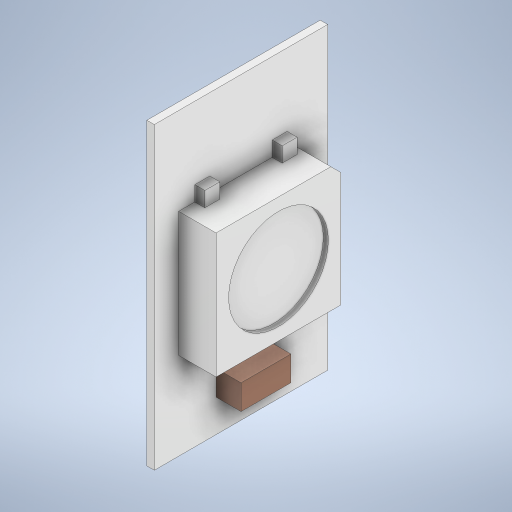
# Autodesk Inventor part: Base144
Saved by Autodesk Inventor 2023 (Build 270158000, 158)
## iProperties
Created: 2024-03-20
Part Number: Base144
Material: Generic
Document SubType Name: Modeling
Designer: noname
Density: 1 g/cm^3
Appearance: Smooth - White
Author: noname
Autodesk Inventor part; units mm, degrees
ref_plane "YZ Plane" through (0, 0, 0) normal (1, 0, 0) x (0, 1, 0)
ref_plane "XZ Plane" through (0, 0, 0) normal (0, 1, 0) x (-1, 0, 0)
ref_plane "XY Plane" through (0, 0, 0) normal (0, 0, 1) x (1, 0, 0)
sketch "Sketch1" plane through (0, 0, 0) normal (1, 0, 0) x (0, 1, 0)
  line L0 (0, 0) -> (12, 0)
  line L1 (12, 0) -> (12, -6.95)
  line L2 (12, -6.95) -> (0, -6.95)
  line L3 (0, -6.95) -> (0, 0)
  dimension "d0" = 12
  dimension "d1" = 6.95
  constraints: 8 end point, 2 parallel, 1 horizontal, 1 perpendicular
  measures "d0" distance between parallel lines of L3 L1
  measures "d1" distance between parallel lines of L2 L0
extrude "Extrusion1" add sketch "Sketch1" along normal blind 0.3
sketch "Sketch2" plane through (0.3, 0, 0) normal (1, 0, 0) x (0, 0, -1)
  line L0 (0.975, 3.5) -> (5.975, 3.5)
  line L1 (5.975, 3.5) -> (5.975, 8.5)
  line L2 (5.975, 8.5) -> (0.975, 8.5)
  line L3 (0.975, 8.5) -> (0.975, 3.5)
  line L4 (6.95, 12) -> (0, 12) projected
  line L5 (6.95, 0) -> (6.95, 12) projected
  point P0 (0, 0)
  point P1 (3.475, 8.5)
  point P2 (3.475, 12)
  point P3 (5.975, 6)
  point P4 (6.95, 6)
  dimension "d4" = 5
  dimension "d5" = 5
  constraints: 8 end point, 4 midpoint, 2 parallel, 1 horizontal, 1 horizontal alignment, 1 perpendicular, 1 vertical alignment
  measures "d4" distance between parallel lines of L1 L3
  measures "d5" distance between parallel lines of L0 L2
extrude "Extrusion2" add sketch "Sketch2" along normal blind 1.5
sketch "Sketch3" plane through (1.8, 0, 0) normal (1, 0, 0) x (0, 0, -1)
  circle A0 centre (3.475, 6) radius 2
  line L0 (0.975, 3.5) -> (5.975, 3.5) projected
  line L1 (5.975, 3.5) -> (5.975, 8.5) projected
  point P0 (0, 0)
  point P1 (3.475, 3.5)
  point P2 (5.975, 6)
  dimension "d8" = 4
  constraints: 2 midpoint, 1 centre point, 1 horizontal alignment, 1 vertical alignment
  measures "d8" diameter of A0
extrude "Extrusion3" cut sketch "Sketch3" against normal blind 0.2
chamfer "Chamfer1" distance 0.4 angle 45 1 edges at (1.05, 8.5, -5.975)
sketch "Sketch5" plane through (0.3, 0, 0) normal (1, 0, 0) x (0, 0, -1)
  line L0 (5.975, 3.5) -> (0.975, 3.5) projected
  line L1 (1.625, 3.5) -> (2.225, 3.5)
  line L2 (2.225, 3.5) -> (2.225, 2.9)
  line L3 (2.225, 2.9) -> (1.625, 2.9)
  line L4 (1.625, 2.9) -> (1.625, 3.5)
  line L5 (0.975, 3.5) -> (0.975, 8.5) projected
  line L6 (0.975, 6) -> (5.975, 6)
  line L7 (5.975, 8.1) -> (5.975, 3.5) projected
  line L8 (3.475, 3.5) -> (3.475, 8.5)
  line L9 (0.975, 8.5) -> (5.575, 8.5) projected
  line L10 (5.325, 3.5) -> (4.725, 3.5)
  line L11 (4.725, 3.5) -> (4.725, 2.9)
  line L12 (4.725, 2.9) -> (5.325, 2.9)
  line L13 (5.325, 2.9) -> (5.325, 3.5)
  line L14 (1.625, 8.5) -> (2.225, 8.5)
  line L15 (2.225, 8.5) -> (2.225, 9.1)
  line L16 (2.225, 9.1) -> (1.625, 9.1)
  line L17 (1.625, 9.1) -> (1.625, 8.5)
  line L18 (5.325, 8.5) -> (4.725, 8.5)
  line L19 (4.725, 8.5) -> (4.725, 9.1)
  line L20 (4.725, 9.1) -> (5.325, 9.1)
  line L21 (5.325, 9.1) -> (5.325, 8.5)
  point P0 (0, 0)
  dimension "d14" = 0.6
  dimension "d15" = 0.6
  dimension "d16" = 2.5
  constraints: 36 end point, 12 symmetric about line, 3 point on line, 2 horizontal, 2 midpoint, 2 parallel, 1 perpendicular, 1 vertical
  measures "d14" distance between parallel lines of L0 L3
  measures "d15" distance between parallel lines of L2 L4
  measures "d16" diameter of L2 L8
extrude "Extrusion4" add sketch "Sketch5" along normal blind 0.4 contours L13 L12 L11 L0 | L2 L3 L4 L0 | L9 L17 L16 L15 | L19 L20 L21 L9
sketch "Sketch6" plane through (0.3, 0, 0) normal (1, 0, 0) x (0, 0, -1)
  line L0 (2.475, 1.3) -> (4.475, 1.3)
  line L1 (4.475, 1.3) -> (4.475, 2.3)
  line L2 (4.475, 2.3) -> (2.475, 2.3)
  line L3 (2.475, 2.3) -> (2.475, 1.3)
  line L4 (0, 0) -> (6.95, 0) projected
  point P0 (3.475, 1.3)
  point P1 (3.475, 0)
  dimension "d19" = 1
  dimension "d20" = 2
  dimension "d21" = 1.3
  constraints: 8 end point, 2 midpoint, 2 parallel, 1 horizontal, 1 perpendicular, 1 vertical alignment
  measures "d19" distance between parallel lines of L0 L2
  measures "d20" distance between parallel lines of L3 L1
  measures "d21" distance between parallel lines of L4 L0
extrude "Extrusion5" add sketch "Sketch6" along normal blind 1
body "Solid1"
